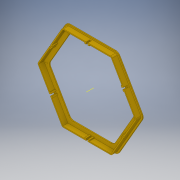
# Autodesk Inventor part: Cover v1
Saved by Autodesk Inventor 2019 (Build 230136000, 136)
## iProperties
Created: 2021-07-14
Part Number: Cover v1
Material: Generic
Document SubType Name: Modeling
Designer: Lix
Density: 1 g/cm^3
Appearance: Gold
d0: 175,000 mm
d1: 2,000 mm
d2: 0,00 deg
d15: 3,000 mm
d16: 2,000 mm
d17: 10,000 mm
d18: 0,00 deg
d19: 8,000 mm
d20: 7,000 mm
d21: 0,00 deg
d22: 10,000 mm
d23: 4,000 mm
d24: 10,000 mm
d25: 3,300 mm
d26: 7,500 mm
d27: 0,00 deg
d28: 4,000 mm
d29: 3,000 mm
d31: 0,00 deg
d32: 6,000 ul
d33: 360,00 deg
Author: Lix
Autodesk Inventor part; units mm, degrees
ref_plane "YZ Plane" through (0, 0, 0) normal (1, 0, 0) x (0, 1, 0)
ref_plane "XZ Plane" through (0, 0, 0) normal (0, 1, 0) x (-1, 0, 0)
ref_plane "XY Plane" through (0, 0, 0) normal (0, 0, 1) x (1, 0, 0)
sketch "Sketch1" plane through (0, 0, 0) normal (0, 0, 1) x (1, 0, 0)
  line L0 (50.5181, -87.5) -> (-50.5181, -87.5)
  line L1 (-50.5181, -87.5) -> (-101.0363, 0)
  line L2 (-101.0363, 0) -> (-50.5181, 87.5)
  line L3 (-50.5181, 87.5) -> (50.5181, 87.5)
  line L4 (50.5181, 87.5) -> (101.0363, 0)
  line L5 (101.0363, 0) -> (50.5181, -87.5)
  point P0 (0, 0)
  point P1 (0, 0)
  dimension "d0" = 175
  constraints: 12 end point, 1 coincident, 1 horizontal, 13 other
  measures "d0" distance between parallel lines of L4 L1
extrude "Extrusion1" add sketch "Sketch1" along normal blind 2
sketch "Sketch5" plane through (0, 0, 2) normal (0, 0, 1) x (1, 0, 0)
  line L0 (-50.5181, -87.5) -> (50.5181, -87.5) projected
  line L1 (50.5181, -87.5) -> (101.0363, 0) projected
  line L2 (101.0363, 0) -> (50.5181, 87.5) projected
  line L3 (50.5181, 87.5) -> (-50.5181, 87.5) projected
  line L4 (-50.5181, 87.5) -> (-101.0363, 0) projected
  line L5 (-101.0363, 0) -> (-50.5181, -87.5) projected
  line L6 (-97.5722, 0) -> (-48.7861, 84.5)
  line L7 (-48.7861, 84.5) -> (48.7861, 84.5)
  line L8 (48.7861, 84.5) -> (97.5722, 0)
  line L9 (97.5722, 0) -> (48.7861, -84.5)
  line L10 (48.7861, -84.5) -> (-48.7861, -84.5)
  line L11 (-48.7861, -84.5) -> (-97.5722, 0)
  line L12 (-95.2628, 0) -> (-47.6314, 82.5)
  line L13 (-47.6314, 82.5) -> (47.6314, 82.5)
  line L14 (47.6314, 82.5) -> (95.2628, 0)
  line L15 (95.2628, 0) -> (47.6314, -82.5)
  line L16 (47.6314, -82.5) -> (-47.6314, -82.5)
  line L17 (-47.6314, -82.5) -> (-95.2628, 0)
  point P0 (0, 0)
  dimension "d15" = 3
  dimension "d16" = 2
  constraints: 24 end point, 10 other
  measures "d15" distance between parallel lines of L4 L6
  measures "d16" distance between parallel lines of L11 L17
extrude "Extrusion5" add sketch "Sketch5" along normal blind 10 contours L6 L7 L8 L9 L10 L11
sketch "Sketch7" plane through (0, 0, 2) normal (0, 0, 1) x (1, 0, 0)
  line L0 (47.6314, 82.5) -> (-47.6314, 82.5) projected
  line L1 (-47.6314, 82.5) -> (-95.2628, 0) projected
  line L2 (-95.2628, 0) -> (-47.6314, -82.5) projected
  line L3 (-47.6314, -82.5) -> (47.6314, -82.5) projected
  line L4 (47.6314, -82.5) -> (95.2628, 0) projected
  line L5 (95.2628, 0) -> (47.6314, 82.5) projected
  line L6 (-43.0126, -74.5) -> (-86.0252, 0)
  line L7 (-86.0252, 0) -> (-43.0126, 74.5)
  line L8 (-43.0126, 74.5) -> (43.0126, 74.5)
  line L9 (43.0126, 74.5) -> (86.0252, 0)
  line L10 (86.0252, 0) -> (43.0126, -74.5)
  line L11 (43.0126, -74.5) -> (-43.0126, -74.5)
  point P0 (0, 0)
  dimension "d19" = 8
  constraints: 12 end point, 5 other
  measures "d19" distance between parallel lines of L2 L6
extrude "Extrusion6" cut sketch "Sketch7" against normal blind 7 contours L6 L7 L8 L9 L10 L11
fillet "Fillet1" radius 10 6 edges at (50.5181, 87.5, 1) (101.0363, 0, 1) (50.5181, -87.5, 1) (-50.5181, -87.5, 1) (-101.0363, 0, 1) (-50.5181, 87.5, 1)
fillet "Fillet1" radius 4 6 edges at (-97.5722, 0, 7) (-48.7861, 84.5, 7) (48.7861, 84.5, 7) (97.5722, 0, 7) (-48.7861, -84.5, 7) (48.7861, -84.5, 7)
fillet "Fillet2" radius 10 6 edges at (43.0126, -74.5, 1) (86.0252, 0, 1) (43.0126, 74.5, 1) (-43.0126, 74.5, 1) (-86.0252, 0, 1) (-43.0126, -74.5, 1)
sketch "Sketch8" plane through (0, 0, 12) normal (0, 0, 1) x (1, 0, 0)
  line L0 (-1.65, 82.5) -> (1.65, 82.5)
  line L1 (1.65, 82.5) -> (1.65, 84.5)
  line L2 (1.65, 84.5) -> (-1.65, 84.5)
  line L3 (-1.65, 84.5) -> (-1.65, 82.5)
  line L4 (46.4767, 84.5) -> (-46.4767, 84.5) projected
  line L5 (-47.6314, 82.5) -> (47.6314, 82.5) projected
  point P0 (0, 0)
  point P1 (0, 84.5)
  point P2 (0, 84.5)
  point P3 (-45.8993, 83.5)
  point P4 (45.8993, 83.5)
  point P5 (0, 0)
  dimension "d25" = 3.3
  constraints: 8 end point, 2 coincident, 2 horizontal, 2 midpoint, 2 parallel, 1 collinear, 1 perpendicular, 1 other
  measures "d25" distance between parallel lines of L1 L3
extrude "Extrusion7" cut sketch "Sketch8" against normal blind 7.5
sketch "Sketch9" plane through (0, 0, 12) normal (0, 0, 1) x (1, 0, 0)
  line L0 (-4.65, 80.5) -> (-1.65, 80.5)
  line L1 (-1.65, 80.5) -> (-1.65, 84.5)
  line L2 (-1.65, 84.5) -> (-4.65, 84.5)
  line L3 (-4.65, 84.5) -> (-4.65, 80.5)
  line L4 (1.65, 82.5) -> (-1.65, 82.5) projected
  line L5 (1.65, 84.5) -> (1.65, 82.5) projected
  line L6 (-1.65, 84.5) -> (1.65, 84.5) projected
  line L7 (-1.65, 82.5) -> (-1.65, 84.5) projected
  line L8 (0, 82.5) -> (0, 81.6202) construction
  line L9 (1.65, 82.5) -> (-1.65, 82.5) projected
  line L10 (-1.65, 82.5) -> (-1.65, 84.5) projected
  line L11 (4.65, 80.5) -> (1.65, 80.5)
  line L12 (1.65, 80.5) -> (1.65, 84.5)
  line L13 (1.65, 84.5) -> (4.65, 84.5)
  line L14 (4.65, 84.5) -> (4.65, 80.5)
  line L15 (-1.65, 84.5) -> (-46.4767, 84.5) projected
  point P0 (0, 0)
  point P1 (-45.8993, 83.5)
  dimension "d28" = 4
  dimension "d29" = 3
  constraints: 18 end point, 5 symmetric about line, 2 collinear, 2 parallel, 1 horizontal, 1 midpoint, 1 perpendicular, 1 vertical, 1 other
  measures "d28" distance of L2.end L0.start
  measures "d29" distance of L1.end L2.end
extrude "Extrusion8" add sketch "Sketch9" against normal up to surface (10 mm away) contours L3 L2 L1 L0 | L5 L13 L14 L11 L12
pattern_circular "Circular Pattern1" count 6 over 360 about axis through (0, 0, 0) along (0, 0, 1) of "Extrusion8", "Extrusion7"
sketch "Sketch11" plane through (0, 0, 2) normal (0, 0, 1) x (1, 0, 0)
  circle A0 centre (-91.3063, 0) radius 0.5
  circle A1 centre (-88.3063, 0) radius 0.5
  point P0 (0, 0)
  point P1 (-95.2628, 0)
  dimension "d35" = 1
  dimension "d36" = 3
  constraints: 2 centre point, 2 horizontal alignment, 1 equal radius
  measures "d35" diameter of A0
  measures "d36" distance of A1.centre A0.centre
extrude "Extrusion9" cut sketch "Sketch11" against normal blind 0.5
body "Solid1"
